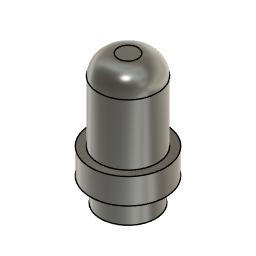
light-pipe (Autodesk Fusion 360 design; units mm, degrees)
Autodesk Fusion 360 part; units mm, degrees
sketch "drawing" plane through (0, 0, 0) normal (1, 0, 0) x (0, 1, 0)
  line L0 (0, 4.1) -> (0.5, 4.1)
  line L1 (1.5, 3.1) -> (1.5, 0)
  line L2 (0, 0) -> (0, 4.1)
  line L3 (1.75, 0) -> (22.5, 0)
  line L4 (0, 1.75) -> (0, 22.5)
  arc A0 (1.5, 3.1) -> (0.5, 4.1) centre (0.5, 3.1) ccw
  line L5 (1.5, 0) -> (1.9, 0)
  line L6 (1.9, 0) -> (1.9, -1.3)
  line L7 (1.9, -1.3) -> (1.4, -1.3)
  line L8 (0, -1.3) -> (0, 0)
  line L9 (20, 0) -> (2.5, 0)
  line L10 (1.4, -1.3) -> (1.4, -2.5)
  line L11 (1.4, -2.5) -> (0, -2.5)
  line L12 (0, -2.5) -> (0, -1.3)
  dimension "d1" = 1.5
  dimension "d3" = 1
  dimension "d4" = 1.9
  dimension "d5" = 1.3
  dimension "d6" = 4.1
  dimension "d7" = 1.4
  dimension "d8" = 2.5
  constraint horizontal L0
  constraint vertical L1
  constraint vertical L2
  constraint collinear L2 L4
  constraint tangent L0 A0
  constraint tangent L1 A0
  constraint horizontal L5
  constraint vertical L6
  constraint horizontal L7
  constraint vertical L8
  constraint coincident L2.start L8.end
  constraint vertical L10
  constraint horizontal L11
  constraint vertical L12
  constraint collinear L3 L5
  measures "d1" distance of L2.start L1
  measures "d3" radius of A0
  measures "d4" distance of L6 L8
  measures "d5" distance of L5 L7
  measures "d6" distance of L0 L9
  measures "d7" distance of L10 L12
  measures "d8" distance of L5 L11
revolve "Revolve1" add sketch "drawing" angle 360 about axis through (0, 0, 0) along (0, 0, 1)
